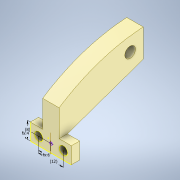
# Autodesk Inventor part: motor_elytra_interface
Saved by Autodesk Inventor 2021 (Build 250183000, 183)
## iProperties
Created: 2020-11-22
Part Number: motor_elytra_interface
Material: Nylon 6/6
Document SubType Name: Modeling
Designer: Paco
Density: 1.13 g/cm^3
Appearance: Nylon 6
Mass: 6.3153 g
Surface Area: 28.3041 cm^2
Volume: 5.58876 cm^3
Author: Paco
Autodesk Inventor part; units mm, degrees
ref_plane "YZ Plane" through (0, 0, 0) normal (1, 0, 0) x (0, 1, 0)
ref_plane "XZ Plane" through (0, 0, 0) normal (0, 1, 0) x (-1, 0, 0)
ref_plane "XY Plane" through (0, 0, 0) normal (0, 0, 1) x (1, 0, 0)
sketch "Sketch1" plane through (0, 0, 0) normal (0, 0, 1) x (1, 0, 0)
  line L0 (-8.802, 2.3397) -> (11.198, 2.3397)
  line L1 (11.198, 2.3397) -> (11.198, -5.6603)
  line L2 (11.198, -5.6603) -> (-8.802, -5.6603)
  line L3 (-8.802, -5.6603) -> (-8.802, 2.3397)
  circle A0 centre (-4.802, -1.6603) radius 2
  circle A1 centre (7.198, -1.6603) radius 2
  point P0 (0, 0)
  dimension "d4" = 4
  dimension "d0" = 4
  dimension "d1" = 4
  dimension "d2" = 12
  dimension "d3" = 4
  dimension "d5" = 4
  dimension "d7" = 8
  dimension "d8" = 4
  dimension "d9" = 20
  dimension "d10" = 4
  constraints: 8 end point, 2 centre point, 2 parallel, 1 horizontal, 1 perpendicular
  measures "d0" diameter of A0
  measures "d1" diameter of A1
  measures "d2" distance of A1.centre A0.centre
  measures "d3" distance from line of L0 A0.centre
  measures "d5" distance from line of L2 A1.centre
  measures "d7" distance between parallel lines of L2 L0
  measures "d8" distance from line of L2 A0.centre
  measures "d9" distance of L0.start L0.end
  measures "d10" distance from line of L3 A0.centre
extrude "Extrusion1" add sketch "Sketch1" along normal blind 4
ref_plane "Work Plane1" through (1.198, -5.6603, 0) normal (1, 0, 0) x (0, 0, -1)
sketch "Sketch2" plane through (1.198, -5.6603, 0) normal (1, 0, 0) x (0, 0, -1)
  arc A0 (36.9246, 34.6197) -> (-4, 21) centre (41.9479, -48.7697) ccw
  line L0 (0, 0) -> (0, 8) projected
  line L1 (36.9247, 21) -> (36.9246, 34.6197)
  arc A1 (44.549, 70.6711) -> (-44.2597, 70.8526) centre (0, 0) ccw
  circle A2 centre (9.9821, 76.8133) radius 2.6
  line L2 (9.9821, 96.2846) -> (9.9821, 47.2392) construction
  line L3 (62.1306, 76.8133) -> (-24.9977, 76.8133) construction
  line L4 (0, 0) -> (0, 8) construction
  circle A3 centre (30.5669, 27.142) radius 2.6
  line L5 (-4, 0) -> (-4, 8) projected
  line L6 (0, 8) -> (-4, 8) projected
  line L7 (36.9247, 21) -> (0, 8)
  line L8 (0, 8) -> (-4, 8)
  line L9 (36.9247, 21) -> (-4, 21) construction
  line L10 (-4, 21) -> (-4, 8)
  point P0 (0, 5.6603)
  dimension "d15" = 34.5669
  dimension "d16" = 6.1422
  dimension "d17" = 34.5669
  dimension "d22" = 13.6197
  dimension "d27" = 5.2
  dimension "d32" = 6.142
  dimension "d33" = 13
  constraints: 16 end point, 4 centre point, 4 point on circle, 3 vertical, 2 horizontal, 1 coincident, 1 collinear
  measures "d15" distance from line of L2 A1.start
  measures "d16" distance from line of A1.start L3
  measures "d17" horizontal distance of L5.end point (30.567, 27.142)
  measures "d22" distance of L1.start L1.end
  measures "d27" diameter of A3
  measures "d32" distance from line of L9 point (30.567, 27.142)
  measures "d33" distance of L9.end L5.end
extrude "Extrusion4" add sketch "Sketch2" along normal mid plane 8 contours L1 L7 L6 L10 A0
sketch "Sketch3" plane through (0, 0, 4) normal (0, 0, 1) x (1, 0, 0)
  circle A0 centre (7.198, -1.6603) radius 2 projected
  circle A1 centre (-4.802, -1.6603) radius 2 projected
  line L0 (-8.802, 2.3397) -> (-8.802, -5.6603) projected
  line L1 (-8.802, -5.6603) -> (11.198, -5.6603) projected
  circle A2 centre (1.198, -1.6603) radius 0.6445
  point P0 (0, 0)
  dimension "d28" = 12
  dimension "d29" = 6
  dimension "d30" = 8
  dimension "d31" = 4
  constraints: 1 centre point, 1 coincident
  measures "d28" distance of A0.centre A1.centre
  measures "d29" distance of point (1.198, -1.66) A1.centre
  measures "d30" distance of L0.start L0.end
  measures "d31" distance from line of L1 point (1.198, -1.66)
equation "\"d4\" = d3"
equation "\"d3\" = d8"
equation "\"d5\" = d4"
equation "\"d29\" = 0.5 * d28"
equation "\"d31\" = 0.5 * d30"
body "Solid1"
